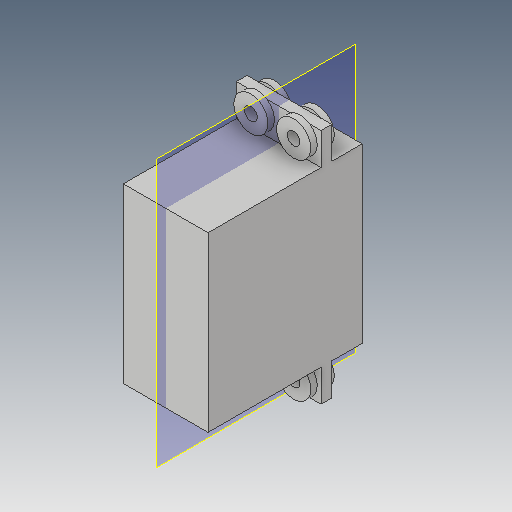
# Autodesk Inventor part: Part100
Saved by Autodesk Inventor 2019.4 (Build 234330000, 330)
## iProperties
Created: 2018-08-29
Part Number: Part100
Material: 一般
Document SubType Name: Modeling
Designer: AzLIer
Density: 1 g/cm^3
Appearance: 既定
Author: AzLIer
Autodesk Inventor part; units mm, degrees
sketch "スケッチ1" plane through (0, 0, 0) normal (0, 0, 1) x (1, 0, 0)
  line L0 (9.9, -20.2) -> (-9.9, -20.2)
  line L1 (-9.9, -20.2) -> (-9.9, 20.2)
  line L2 (-9.9, 20.2) -> (9.9, 20.2)
  line L3 (9.9, 20.2) -> (9.9, -20.2)
  line L4 (9.9, -20.2) -> (-9.9, 20.2) construction
  line L5 (-9.9, -20.2) -> (9.9, 20.2) construction
  circle A0 centre (-10.932, 25.3443) radius 2.25
  point P0 (0, 0)
  dimension "d0" = 4.5
  dimension "d1" = 40.4
  dimension "d2" = 19.8
  constraints: 12 end point, 2 midpoint, 2 parallel, 1 centre point, 1 horizontal, 1 perpendicular
  measures "d0" diameter of A0
  measures "d1" distance of L0.end L1.end
  measures "d2" distance of L1.end L2.end
extrude "押し出し1" add sketch "スケッチ1" along normal blind 36 contours L0 L1 L2 L3
sketch "スケッチ2" plane through (0, 0, 0) normal (0, 0, -1) x (-1, 0, 0)
  circle A0 centre (0, 10.2) radius 3
  line L0 (9.9, 20.2) -> (-9.9, 20.2) projected
  point P0 (0, 0)
  dimension "d5" = 6
  dimension "d6" = 10
  constraints: 1 centre point, 1 vertical alignment
  measures "d5" diameter of A0
  measures "d6" distance from line of A0.centre L0
extrude "押し出し2" add sketch "スケッチ2" along normal blind 6.2
ref_plane "作業平面1" through (0, 0, 9.6) normal (0, 0, 1) x (1, 0, 0)
sketch "スケッチ4" plane through (0, 0, 9.6) normal (0, 0, 1) x (1, 0, 0)
  line L0 (-9.9, -20.2) -> (9.9, -20.2) projected
  line L1 (9.9, -20.2) -> (9.9, 20.2) projected
  line L2 (9.9, 20.2) -> (-9.9, 20.2) projected
  line L3 (-9.9, 20.2) -> (-9.9, -20.2) projected
  line L4 (-9.9, 20.2) -> (9.9, 20.2)
  line L5 (9.9, 20.2) -> (9.9, 27.7)
  line L6 (9.9, 27.7) -> (-9.9, 27.7)
  line L7 (-9.9, 27.7) -> (-9.9, 20.2)
  line L8 (-9.9, -20.2) -> (9.9, -20.2)
  line L9 (9.9, -20.2) -> (9.9, -27.7)
  line L10 (9.9, -27.7) -> (-9.9, -27.7)
  line L11 (-9.9, -27.7) -> (-9.9, -20.2)
  circle A0 centre (-5, 24.4) radius 1.5
  circle A1 centre (5, 24.4) radius 1.5
  line L12 (0, 27.7) -> (0, 20.2)
  point P0 (0, 0)
  dimension "d10" = 7.5
  dimension "d11" = 7.5
  dimension "d12" = 3
  dimension "d13" = 4.2
  dimension "d15" = 10
  dimension "d16" = 5
  dimension "d17" = 4.2
  constraints: 18 end point, 4 parallel, 2 centre point, 2 collinear, 2 horizontal, 2 midpoint, 2 perpendicular, 1 equal radius
  measures "d10" distance of L5.end L4.end
  measures "d11" distance of L8.end L9.end
  measures "d12" diameter of A0
  measures "d13" distance from line of L4 A0.centre
  measures "d15" distance of A1.centre A0.centre
  measures "d16" distance from line of L12 A0.centre
  measures "d17" distance from line of L4 A1.centre
extrude "押し出し3" add sketch "スケッチ4" against normal blind 2.5 contours L7 L6 L12 L2 | L2 L12 L6 L5
ref_plane "作業平面2" through (-9.9, 0, 36) normal (0, 1, 0) x (1, 0, 0)
mirror "ミラー1" about plane through (-9.9, 0, 36) normal (0, 1, 0) of "押し出し3"
sketch "スケッチ5" plane through (0, 0, 7.1) normal (0, 0, -1) x (-1, 0, 0)
  circle A0 centre (5, 24.4) radius 1.5 projected
  circle A1 centre (-5, 24.4) radius 1.5 projected
  line L0 (9.9, 20.2) -> (-9.9, 20.2) projected
  line L1 (9.9, 20.2) -> (9.9, 27.7) projected
  line L2 (9.9, 27.7) -> (-9.9, 27.7) projected
  line L3 (-9.9, 27.7) -> (-9.9, 20.2) projected
  circle A2 centre (5, -24.4) radius 1.5 projected
  circle A3 centre (-5, -24.4) radius 1.5 projected
  line L4 (-9.9, -20.2) -> (9.9, -20.2) projected
  line L5 (-9.9, -27.7) -> (-9.9, -20.2) projected
  line L6 (9.9, -27.7) -> (-9.9, -27.7) projected
  line L7 (9.9, -20.2) -> (9.9, -27.7) projected
  circle A4 centre (-5, 24.4) radius 4
  circle A5 centre (5, 24.4) radius 4
  circle A6 centre (-5, -24.4) radius 4
  circle A7 centre (5, -24.4) radius 4
  point P0 (0, 0)
  dimension "d20" = 8
  dimension "d21" = 8
  dimension "d22" = 8
  dimension "d23" = 8
  constraints: 4 centre point, 4 coincident
  measures "d20" diameter of A4
  measures "d21" diameter of A5
  measures "d22" diameter of A6
  measures "d23" diameter of A7
extrude "押し出し4" add sketch "スケッチ5" along normal blind 1.5 contours A5 L2 | L2 A5 | A4 L2 | L2 A4 | A6 L6 | L6 A6 | A7 L6 | L6 A7
ref_plane "作業平面3" through (0, 0, 8.35) normal (0, 0, -1) x (-1, 0, 0)
mirror "ミラー2" about plane through (0, 0, 8.35) normal (0, 0, -1) of "押し出し4"
ref_plane "作業平面4" through (0, -20.2, 0) normal (-1, 0, 0) x (0, 0, 1)
equation "\"d16\" = 0.5 * d15"
equation "\"d17\" = d13"
